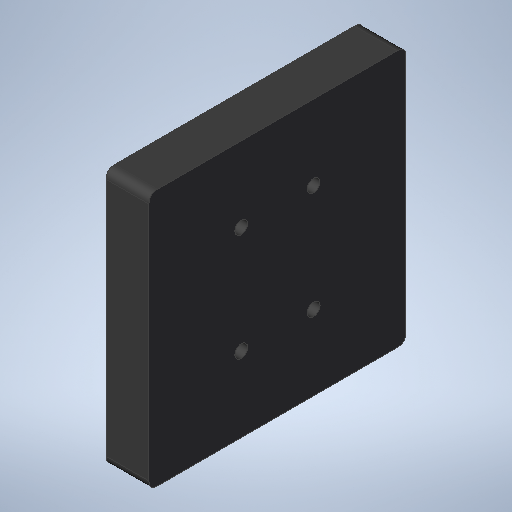
# Autodesk Inventor part: Mount
Saved by Autodesk Inventor 2025.1 (Build 291241000, 241)
## iProperties
Created: 2024-11-09
Part Number: Mount
Material: Generic
Document SubType Name: Modeling
Designer: 13156
Density: 1 g/cm^3
Appearance: Default
Author: 13156
Autodesk Inventor part; units mm, degrees
ref_plane "YZ Plane" through (0, 0, 0) normal (1, 0, 0) x (0, 1, 0)
ref_plane "XZ Plane" through (0, 0, 0) normal (0, 1, 0) x (-1, 0, 0)
ref_plane "XY Plane" through (0, 0, 0) normal (0, 0, 1) x (1, 0, 0)
sketch "Sketch3" plane through (0, 0, 0) normal (1, 0, 0) x (0, 1, 0)
  line L0 (30, 30) -> (-30, 30)
  line L1 (-30, 30) -> (-30, -30)
  line L2 (-30, -30) -> (30, -30)
  line L3 (30, -30) -> (30, 30)
  point P0 (0, 0)
  dimension "d7" = 60
  dimension "d8" = 60
  dimension "d9" = 30
  dimension "d10" = 30
  constraints: 8 end point, 2 parallel, 1 horizontal, 1 perpendicular
  measures "d7" distance of L2.end L0.start
  measures "d8" distance of L1.end L2.end
  measures "d9" distance from line of L2 point (0, 0)
  measures "d10" distance from line of L1 point (0, 0)
extrude "Extrusion2" add sketch "Sketch3" along normal blind 10
fillet "Fillet2" radius 2 4 edges at (5, 30, -30) (5, 30, 30) (5, -30, -30) (5, -30, 30) curvature continuous yes
sketch "Sketch4" plane through (10, 0, 0) normal (1, 0, 0) x (0, 0, -1)
  circle A0 centre (-8.45, 12.5) radius 1.5
  circle A1 centre (8.45, 12.5) radius 1.5
  circle A2 centre (8.45, -12.5) radius 1.5
  circle A3 centre (-8.45, -12.5) radius 1.5
  point P0 (0, 0)
  dimension "d14" = 3
  dimension "d15" = 16.9
  dimension "d16" = 8.45
  dimension "d17" = 0
  dimension "d18" = 0
  dimension "d19" = 0
  dimension "d20" = 25
  dimension "d21" = 12.5
  dimension "d22" = 12.5
  constraints: 4 centre point, 3 equal radius
  measures "d14" diameter of A0
  measures "d15" distance of A1.centre A0.centre
  measures "d16" horizontal distance of point (0, 0) A0.centre
  measures "d17" horizontal distance of A3.centre A0.centre
  measures "d18" horizontal distance of A1.centre A2.centre
  measures "d19" vertical distance of A2.centre A3.centre
  measures "d20" distance of A1.centre A2.centre
  measures "d21" vertical distance of point (0, 0) A1.centre
  measures "d22" vertical distance of point (0, 0) A0.centre
extrude "Extrusion3" cut sketch "Sketch4" against normal blind 14.1125
body "Solid2"
